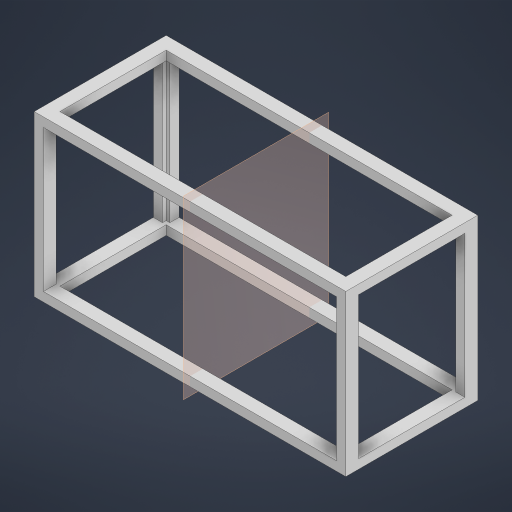
# Autodesk Inventor part: OuterShell
Saved by Autodesk Inventor 2023 (Build 270158000, 158)
## iProperties
Created: 2022-08-22
Part Number: OuterShell
Material: Generic
Document SubType Name: Modeling
Designer: Mike
Density: 1 g/cm^3
Appearance: Default
Author: Mike
Autodesk Inventor part; units mm, degrees
ref_plane "YZ Plane" through (0, 0, 0) normal (1, 0, 0) x (0, 1, 0)
ref_plane "XZ Plane" through (0, 0, 0) normal (0, 1, 0) x (-1, 0, 0)
ref_plane "XY Plane" through (0, 0, 0) normal (0, 0, 1) x (1, 0, 0)
sketch "Sketch1" plane through (0, 0, 0) normal (0, 0, 1) x (1, 0, 0)
  line L0 (0, 0) -> (680, 0)
  line L1 (680, 0) -> (680, 350)
  line L2 (680, 350) -> (0, 350)
  line L3 (0, 350) -> (0, 0)
  line L4 (660, 20) -> (20, 20)
  line L5 (20, 20) -> (20, 330)
  line L6 (20, 330) -> (660, 330)
  line L7 (660, 330) -> (660, 20)
  dimension "d0" = 680
  dimension "d1" = 350
  dimension "d2" = 20
  constraints: 16 end point, 4 perpendicular, 1 horizontal, 1 vertical, 3 other
  measures "d0" distance of L0.start L0.end
  measures "d1" distance of L0.end L1.end
  measures "d2" distance between parallel lines of L0 L4
extrude "Extrusion1" add sketch "Sketch1" against normal blind 28
sketch "Sketch2" plane through (680, 0, 0) normal (1, 0, 0) x (0, 0, -1)
  line L0 (0, 350) -> (28, 350) projected
  line L1 (28, 350) -> (288, 350)
  line L2 (288, 350) -> (288, 0)
  line L3 (28, 350) -> (28, 0) projected
  line L4 (288, 0) -> (28, 0)
  line L5 (28, 330) -> (268, 330)
  line L6 (268, 330) -> (268, 20)
  line L7 (268, 20) -> (28, 20)
  point P0 (0, 0)
  dimension "d5" = 260
  dimension "d6" = 350
  dimension "d7" = 20
  dimension "d8" = 20
  dimension "d9" = 310
  constraints: 12 end point, 4 perpendicular, 2 point on line, 1 horizontal
  measures "d5" distance of L0.end L1.end
  measures "d6" distance of L1.end L2.end
  measures "d7" distance between parallel lines of L5 L1
  measures "d8" distance between parallel lines of L6 L2
  measures "d9" distance between parallel lines of L5 L7
extrude "Extrusion2" add sketch "Sketch2" against normal blind 28 contours L1 L2 L4 L3 L7 L6 L5
ref_plane "Work Plane1" through (0, 0, -144) normal (0, 0, 1) x (1, 0, 0)
mirror "Mirror1" about plane through (0, 0, -144) normal (0, 0, 1) of "Extrusion1"
ref_plane "Work Plane2" through (340, 0, 0) normal (1, 0, 0) x (0, 0, -1)
mirror "Mirror2" about plane through (340, 0, 0) normal (1, 0, 0) of "Extrusion2"
body "Solid1"
